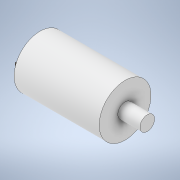
# Autodesk Inventor part: Motor
Saved by Autodesk Inventor 2022 (Build 260153000, 153)
## iProperties
Created: 2022-01-20
Part Number: Motor
Material: Generic
Document SubType Name: Modeling
Designer: 20220
Density: 1 g/cm^3
Appearance: Default
Author: 20220
Autodesk Inventor part; units mm, degrees
ref_plane "YZ Plane" through (0, 0, 0) normal (1, 0, 0) x (0, 1, 0)
ref_plane "XZ Plane" through (0, 0, 0) normal (0, 1, 0) x (-1, 0, 0)
ref_plane "XY Plane" through (0, 0, 0) normal (0, 0, 1) x (1, 0, 0)
sketch "Sketch1" plane through (0, 0, 0) normal (1, 0, 0) x (0, 1, 0)
  circle A0 centre (0, 0) radius 17.78
  dimension "d0" = 35.56
  constraints: 1 centre point, 1 coincident
  measures "d0" diameter of A0
extrude "Extrusion1" add sketch "Sketch1" along normal blind 58.42
sketch "Sketch2" plane through (58.42, 0, 0) normal (1, 0, 0) x (0, 0, -1)
  circle A0 centre (0, 0) radius 5
  dimension "d3" = 10
  constraints: 1 centre point, 1 coincident
  measures "d3" diameter of A0
extrude "Extrusion2" add sketch "Sketch2" along normal blind 15.24
sketch "Sketch3" plane through (0, 0, 0) normal (-1, 0, 0) x (0, 0, 1)
  line L0 (0, 0) -> (-10, 0)
  line L1 (0, 0) -> (10, 0)
  line L2 (10, 2.6452) -> (12, 2.6452)
  line L3 (12, 2.6452) -> (12, -2.3548)
  line L4 (12, -2.3548) -> (10, -2.3548)
  line L5 (10, -2.3548) -> (10, 2.6452)
  line L6 (-10.4235, 2.6452) -> (-12.4235, 2.6452)
  line L7 (-12.4235, 2.6452) -> (-12.4235, -2.3548)
  line L8 (-12.4235, -2.3548) -> (-10.4235, -2.3548)
  line L9 (-10.4235, -2.3548) -> (-10.4235, 2.6452)
  dimension "d6" = 10
  dimension "d7" = 10
  dimension "d8" = 2
  dimension "d9" = 2
  dimension "d10" = 5
  constraints: 20 end point, 4 horizontal, 4 parallel, 2 perpendicular, 2 point on line
  measures "d6" distance of L0.start L0.end
  measures "d7" distance of L0.start L1.end
  measures "d8" distance of L6.start L6.end
  measures "d9" distance of L2.start L2.end
  measures "d10" distance of L6.end L7.end
extrude "Extrusion3" add sketch "Sketch3" along normal blind 5
body "Solid1"
